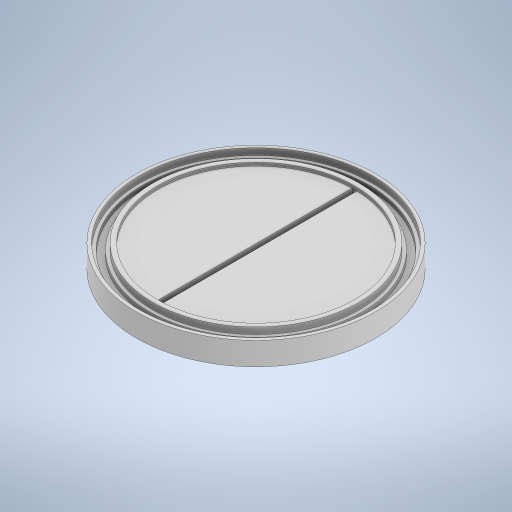
# Autodesk Inventor part: endplate_splitter
Saved by Autodesk Inventor 2023.5 (Build 275446000, 446)
## iProperties
Created: 2025-05-24
Part Number: endplate_splitter
Material: Generic
Document SubType Name: Modeling
Designer: ryanj
Density: 1 g/cm^3
Appearance: Default
Author: ryanj
Autodesk Inventor part; units mm, degrees
ref_plane "YZ Plane" through (0, 0, 0) normal (1, 0, 0) x (0, 1, 0)
ref_plane "XZ Plane" through (0, 0, 0) normal (0, 1, 0) x (-1, 0, 0)
ref_plane "XY Plane" through (0, 0, 0) normal (0, 0, 1) x (1, 0, 0)
sketch "Sketch1" plane through (0, 0, 0) normal (0, 1, 0) x (-1, 0, 0)
  circle A0 centre (0, 0) radius 36.5
  dimension "d0" = 73
  constraints: 1 centre point, 1 coincident
  measures "d0" diameter of A0
extrude "Extrusion1" add sketch "Sketch1" along normal blind 7
sketch "Sketch2" plane through (0, 7, 0) normal (0, 1, 0) x (1, 0, 0)
  circle A0 centre (0, 0) radius 35.5
  circle A1 centre (0, 0) radius 31.5
  dimension "d3" = 71
  dimension "d4" = 63
  constraints: 2 centre point, 2 coincident
  measures "d3" diameter of A0
  measures "d4" diameter of A1
extrude "Extrusion2" cut sketch "Sketch2" against normal blind 2
sketch "Sketch3" plane through (0, 5, 0) normal (0, 1, 0) x (1, 0, 0)
  circle A0 centre (0, 0) radius 34.5
  circle A1 centre (0, 0) radius 32.5
  dimension "d7" = 69
  dimension "d8" = 65
  constraints: 2 centre point, 2 coincident
  measures "d7" diameter of A0
  measures "d8" diameter of A1
extrude "Extrusion3" cut sketch "Sketch3" against normal blind 1.2
sketch "Sketch4" plane through (0, 7, 0) normal (0, 1, 0) x (1, 0, 0)
  circle A0 centre (0, 0) radius 30.085
  dimension "d11" = 60.17
  constraints: 1 centre point, 1 coincident
  measures "d11" diameter of A0
extrude "Extrusion4" cut sketch "Sketch4" against normal blind 1
sketch "Sketch5" plane through (0, 6, 0) normal (0, 1, 0) x (1, 0, 0)
  circle A0 centre (0, 0) radius 30.085 projected
  line L0 (-0.75, -30.0757) -> (0.75, -30.0757)
  line L1 (0.75, -30.0757) -> (0.75, 30.0757)
  line L2 (0.75, 30.0757) -> (-0.75, 30.0757)
  line L3 (-0.75, 30.0757) -> (-0.75, -30.0757)
  line L4 (-0.75, -30.0757) -> (0.75, 30.0757) construction
  line L5 (0.75, -30.0757) -> (-0.75, 30.0757) construction
  dimension "d17" = 1.5
  constraints: 12 end point, 2 midpoint, 2 parallel, 1 horizontal, 1 perpendicular, 1 point on circle
  measures "d17" distance between parallel lines of L1 L3
extrude "Extrusion5" cut sketch "Sketch5" against normal blind 1.5 contours L1 L0 L3 L2
body "Solid1"
